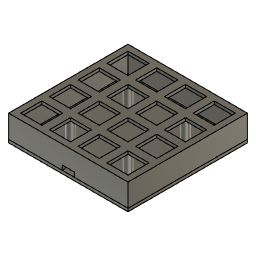
macropad4x4 (Autodesk Fusion 360 design; units mm, degrees)
Autodesk Fusion 360 part; units mm, degrees
sketch "Sketch1" plane through (0, 0, 0) normal (0, 0, 1) x (1, 0, 0)
  line L0 (-4, -4) -> (74.9, -4)
  line L1 (74.9, -4) -> (74.9, 74.9)
  line L2 (74.9, 74.9) -> (-4, 74.9)
  line L3 (-4, 74.9) -> (-4, -4)
  line L4 (0, 0) -> (13.9, 0)
  line L5 (13.9, 0) -> (13.9, 13.9)
  line L6 (13.9, 13.9) -> (0, 13.9)
  line L7 (0, 13.9) -> (0, 0)
  line L8 (19, 13.9) -> (19, 0)
  line L9 (32.9, 13.9) -> (19, 13.9)
  line L10 (32.9, 0) -> (32.9, 13.9)
  line L11 (19, 0) -> (32.9, 0)
  line L12 (38, 13.9) -> (38, 0)
  line L13 (51.9, 13.9) -> (38, 13.9)
  line L14 (51.9, 0) -> (51.9, 13.9)
  line L15 (38, 0) -> (51.9, 0)
  line L16 (57, 13.9) -> (57, 0)
  line L17 (70.9, 13.9) -> (57, 13.9)
  line L18 (70.9, 0) -> (70.9, 13.9)
  line L19 (57, 0) -> (70.9, 0)
  line L20 (0, 32.9) -> (0, 19)
  line L21 (13.9, 32.9) -> (0, 32.9)
  line L22 (13.9, 19) -> (13.9, 32.9)
  line L23 (0, 19) -> (13.9, 19)
  line L24 (19, 32.9) -> (19, 19)
  line L25 (32.9, 32.9) -> (19, 32.9)
  line L26 (32.9, 19) -> (32.9, 32.9)
  line L27 (19, 19) -> (32.9, 19)
  line L28 (38, 32.9) -> (38, 19)
  line L29 (51.9, 32.9) -> (38, 32.9)
  line L30 (51.9, 19) -> (51.9, 32.9)
  line L31 (38, 19) -> (51.9, 19)
  line L32 (57, 32.9) -> (57, 19)
  line L33 (70.9, 32.9) -> (57, 32.9)
  line L34 (70.9, 19) -> (70.9, 32.9)
  line L35 (57, 19) -> (70.9, 19)
  line L36 (0, 51.9) -> (0, 38)
  line L37 (13.9, 51.9) -> (0, 51.9)
  line L38 (13.9, 38) -> (13.9, 51.9)
  line L39 (0, 38) -> (13.9, 38)
  line L40 (19, 51.9) -> (19, 38)
  line L41 (32.9, 51.9) -> (19, 51.9)
  line L42 (32.9, 38) -> (32.9, 51.9)
  line L43 (19, 38) -> (32.9, 38)
  line L44 (38, 51.9) -> (38, 38)
  line L45 (51.9, 51.9) -> (38, 51.9)
  line L46 (51.9, 38) -> (51.9, 51.9)
  line L47 (38, 38) -> (51.9, 38)
  line L48 (57, 51.9) -> (57, 38)
  line L49 (70.9, 51.9) -> (57, 51.9)
  line L50 (70.9, 38) -> (70.9, 51.9)
  line L51 (57, 38) -> (70.9, 38)
  line L52 (0, 70.9) -> (0, 57)
  line L53 (13.9, 70.9) -> (0, 70.9)
  line L54 (13.9, 57) -> (13.9, 70.9)
  line L55 (0, 57) -> (13.9, 57)
  line L56 (19, 70.9) -> (19, 57)
  line L57 (32.9, 70.9) -> (19, 70.9)
  line L58 (32.9, 57) -> (32.9, 70.9)
  line L59 (19, 57) -> (32.9, 57)
  line L60 (38, 70.9) -> (38, 57)
  line L61 (51.9, 70.9) -> (38, 70.9)
  line L62 (51.9, 57) -> (51.9, 70.9)
  line L63 (38, 57) -> (51.9, 57)
  line L64 (57, 70.9) -> (57, 57)
  line L65 (70.9, 70.9) -> (57, 70.9)
  line L66 (70.9, 57) -> (70.9, 70.9)
  line L67 (57, 57) -> (70.9, 57)
  line L68 (-2, -2) -> (72.9, -2)
  line L69 (72.9, -2) -> (72.9, 72.9)
  line L70 (72.9, 72.9) -> (-2, 72.9)
  line L71 (-2, 72.9) -> (-2, -2)
  line L72 (0, 0) -> (70.9, 70.9) construction
  line L73 (0, 70.9) -> (70.9, 0) construction
  line L74 (13.9, 51.9) -> (19, 57) construction
  line L75 (51.9, 57) -> (57, 51.9) construction
  line L76 (57, 19) -> (51.9, 13.9) construction
  line L77 (19, 13.9) -> (13.9, 19) construction
  circle A0 centre (16.45, 16.45) radius 2.5
  circle A1 centre (54.45, 16.45) radius 2.5
  circle A2 centre (54.45, 54.45) radius 2.5
  circle A3 centre (16.45, 54.45) radius 2.5
  circle A4 centre (16.45, 16.45) radius 1
  circle A5 centre (54.45, 16.45) radius 1
  circle A6 centre (54.45, 54.45) radius 1
  circle A7 centre (16.45, 54.45) radius 1
  dimension "d1" = 13.9
  dimension "d4" = 19
  dimension "d5" = 19
  dimension "d6" = 4
  dimension "d7" = 4
  dimension "d8" = 4
  dimension "d9" = 4
  dimension "d12" = 2
  dimension "d13" = 2
  dimension "d14" = 2
  dimension "d15" = 2
  dimension "d18" = 5
  dimension "d19" = 2
  constraint horizontal L0
  constraint vertical L1
  constraint horizontal L2
  constraint vertical L3
  constraint horizontal L4
  constraint vertical L5
  constraint horizontal L6
  constraint vertical L7
  constraint coincident L4.start L7.end
  constraint equal L4 L7
  constraint horizontal L68
  constraint vertical L69
  constraint horizontal L70
  constraint vertical L71
  constraint midpoint L77 A0.centre
  constraint midpoint L76 A1.centre
  constraint midpoint L75 A2.centre
  constraint midpoint L74 A3.centre
  constraint equal A0 A1
  constraint equal A1 A2
  constraint equal A2 A3
  constraint concentric A0 A4
  constraint concentric A1 A5
  constraint concentric A2 A6
  constraint concentric A3 A7
  constraint equal A6 A7
  constraint equal A5 A6
  constraint equal A4 A5
  measures "d1" distance of L4.start L4.end
  measures "d6" distance of L3 L7
  measures "d7" distance of L0 L4
  measures "d8" distance of L2 L65
  measures "d9" distance of L1 L66
  measures "d12" distance of L3 L71
  measures "d13" distance of L0 L68.start
  measures "d14" distance of L2 L70
  measures "d15" distance of L1 L69
  measures "d18" diameter of A0
  measures "d19" diameter of A4
extrude "Extrude1" add sketch "Sketch1" along normal blind 2 contours L0 L1 L2 L3 | L68 L69 L70 L71 | A0 | A1 | A2 | A3 | A4 | A5 | A6 | A7 makes body 1
extrude "Extrude2" add sketch "Sketch1" against normal blind 13 contours L0 L1 L2 L3 bodies 1
extrude "Extrude3" add sketch "Sketch1" against normal up to surface (13 mm away) contours A0 | A1 | A2 | A3 bodies 1
sketch "Sketch2" plane through (0, -2, 0) normal (0, 1, 0) x (-1, 0, 0)
  line L0 (2, 0) -> (-72.9, 0)
  line L1 (-72.9, 0) -> (-72.9, -13)
  line L2 (-72.9, -13) -> (2, -13)
  line L3 (2, -13) -> (2, 0)
  line L4 (-39.45, -13) -> (-31.45, -13)
  line L5 (-31.45, -13) -> (-31.45, -10)
  line L6 (-31.45, -10) -> (-39.45, -10)
  line L7 (-39.45, -10) -> (-39.45, -13)
  line L8 (-74.9, -13) -> (4, 2) construction
  line L9 (-35.45, -5.5) -> (-35.45, -10) construction
  point P0 (4, 2)
  point P1 (-74.9, -13)
  dimension "d22" = 8
  dimension "d23" = 3
  constraint horizontal L4
  constraint vertical L5
  constraint horizontal L6
  constraint vertical L7
  constraint midpoint L8 L9.start
  constraint midpoint L6 L9.end
  constraint vertical L9
  constraint coincident P0 L8.end
  constraint coincident P1 L8.start
  constraint collinear L2 L4
  measures "d22" distance of L4.start L4.end
  measures "d23" distance of L4.end L5.end
extrude "Extrude4" cut sketch "Sketch2" against normal blind 5 contours L2 L4 L5 L6 L7 bodies 1
sketch "Sketch1 (2)" plane through (0, 0, -13) normal (0, 0, -1) x (1, 0, 0) in component "Component"
  line L0 (39.45, 4) -> (39.45, 2)
  line L1 (39.45, 2) -> (72.9, 2)
  line L2 (72.9, 2) -> (72.9, -72.9)
  line L3 (72.9, -72.9) -> (-2, -72.9)
  line L4 (-2, -72.9) -> (-2, 2)
  line L5 (-2, 2) -> (31.45, 2)
  line L6 (31.45, 2) -> (31.45, 4)
  line L7 (31.45, 4) -> (-4, 4)
  line L8 (-4, 4) -> (-4, -74.9)
  line L9 (-4, -74.9) -> (74.9, -74.9)
  line L10 (74.9, -74.9) -> (74.9, 4)
  line L11 (74.9, 4) -> (39.45, 4)
  line L12 (-4, 4) -> (74.9, 4)
  line L13 (74.9, 4) -> (74.9, -74.9)
  line L14 (74.9, -74.9) -> (-4, -74.9)
  line L15 (-4, -74.9) -> (-4, 4)
  circle A0 centre (16.45, -16.45) radius 1 construction
  circle A1 centre (54.45, -16.45) radius 1 construction
  circle A2 centre (54.45, -54.45) radius 1 construction
  circle A3 centre (16.45, -54.45) radius 1 construction
  circle A4 centre (16.45, -16.45) radius 2.5 construction
  circle A5 centre (54.45, -16.45) radius 2.5 construction
  circle A6 centre (54.45, -54.45) radius 2.5 construction
  circle A7 centre (16.45, -54.45) radius 2.5 construction
  circle A8 centre (16.45, -16.45) radius 1 construction
  constraint horizontal L12
  constraint vertical L13
  constraint horizontal L14
  constraint vertical L15
  constraint coincident L9.end L10.start
  constraint coincident L7.end L8.start
  constraint concentric A0 A4
  constraint concentric A1 A5
  constraint concentric A2 A6
  constraint concentric A3 A7
  constraint equal A0 A1
  constraint equal A1 A2
  constraint equal A2 A3
  constraint equal A0 A8
extrude "Extrude1'" add sketch "Sketch1 (2)" along normal blind 2 separate body makes body 2 in component "Component"
sketch "Sketch2 (2)" plane through (0, 0, -15) normal (0, 0, -1) x (1, 0, 0) in component "Component"
  line L0 (-4, -74.9) -> (74.9, -74.9)
  line L1 (74.9, -74.9) -> (74.9, 4)
  line L2 (74.9, 4) -> (-4, 4)
  line L3 (-4, 4) -> (-4, -74.9)
  circle A0 centre (16.45, -16.45) radius 2.5634 construction
  circle A1 centre (54.45, -16.45) radius 1.0382 construction
  circle A2 centre (54.45, -54.45) radius 4.154 construction
  circle A3 centre (16.45, -54.45) radius 3.4752 construction
  circle A4 centre (16.45, -54.45) radius 1 construction
  circle A5 centre (54.45, -54.45) radius 1 construction
  circle A6 centre (54.45, -16.45) radius 1 construction
  circle A7 centre (16.45, -16.45) radius 1 construction
  constraint concentric A3 A4
  constraint concentric A2 A5
  constraint concentric A1 A6
  constraint concentric A0 A7
hole "Hole1" at (16.45, 16.45, -15) at (54.45, 16.45, -15) at (54.45, 54.45, -15) at (16.45, 54.45, -15) direction (0, 0, 1) diameter 2 depth 4 tip angle 118 countersink diameter 5 countersink angle 90 bodies 2 in component "Component"
component "Component" placed x (1, 0, 0) y (0, 1, 0) z (0, 0, 1) at (0, 0, 0)
equation "d6 = d7"
equation "d8 = d7"
equation "d9 = d7"
